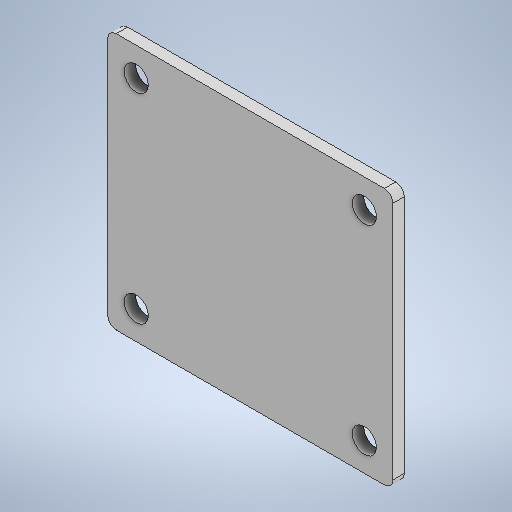
# Autodesk Inventor part: Сrane plate 6
Saved by Autodesk Inventor 2025 (Build 290162010, 162A)
## iProperties
Created: 2024-06-15
Part Number: Сrane plate 6
Material: Generic
Document SubType Name: Sheet Metal
Designer: admin
Density: 1 g/cm^3
Sheet Metal Rule: Default
Appearance: Default
Stock Number: Кран плата 6
Flat Pattern Width: 18 cm
Flat Pattern Length: 20 cm
Flat Pattern Area: 360 cm^2
Sheet Metal Width: 180,000 mm
Sheet Metal Length: 200,000 mm
Sheet Metal Area: 36000,000 mm^2
Author: admin
Autodesk Inventor part; units mm, degrees
ref_plane "YZ Plane" through (0, 0, 0) normal (1, 0, 0) x (0, 1, 0)
ref_plane "XZ Plane" through (0, 0, 0) normal (0, 1, 0) x (-1, 0, 0)
ref_plane "XY Plane" through (0, 0, 0) normal (0, 0, 1) x (1, 0, 0)
sketch "Sketch1" plane through (0, 0, 0) normal (0, 1, 0) x (-1, 0, 0)
  line L0 (100, 90) -> (-100, 90)
  line L1 (-100, 90) -> (-100, -90)
  line L2 (-100, -90) -> (100, -90)
  line L3 (100, -90) -> (100, 90)
  point P0 (0, 0)
  point P1 (0, 90)
  point P2 (100, 0)
  dimension "d0" = 200
  dimension "d1" = 180
  measures "d0" distance of L0.start L0.end
  measures "d1" distance of L2.end L0.start
extrude "Plate1" add sketch "Sketch1" along normal blind 8
sketch "Sketch2" plane through (0, 0, 0) normal (0, -1, 0) x (1, 0, 0)
  line L0 (80, 70) -> (80, -70) construction
  line L1 (-100, -90) -> (-100, 90) projected
  line L2 (100, 90) -> (100, -90) projected
  point P0 (0, 0)
  point P1 (80, 0)
  point P2 (-100, 0)
  dimension "d10" = 20
  dimension "d12" = 20
  constraints: 2 end point, 1 coincident, 1 horizontal alignment, 1 midpoint, 1 vertical, 2 other
  measures "d10" distance between parallel lines of L2 L0
  measures "d12" horizontal distance of L0.start L2.start
hole "Hole1" at (80, 0, 70) at (80, 0, -70) direction (0, 1, 0) diameter 17 end through all
fillet "Corner Round1" radius 6 4 edges at (100, 4, 90) (100, 4, -90) (-100, 4, -90) (-100, 4, 90)
mirror "Mirror1" about plane through (0, 0, 0) normal (1, 0, 0) of "Hole1"
equation "\"d12\" = d10"
equation "\"d8\" = Thickness"
equation "\"d2\" = Thickness"
equation "\"BendRadius\" = Thickness"
equation "\"BendReliefWidth\" = Thickness"
equation "\"BendReliefDepth\" = 0.5 * Thickness"
equation "\"CornerReliefSize\" = 4 * Thickness"
equation "\"MinimumRemnant\" = 2 * Thickness"
equation "\"TransitionRadius\" = BendRadius"
equation "\"JacobiRadiusSize\" = BendRadius"
equation "\"GapSize\" = Thickness"
equation "\"Thickness\" = 8"
body "Solid1"
